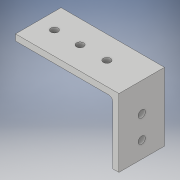
# Autodesk Inventor part: Right_BracketMount
Saved by Autodesk Inventor 2019 (Build 230136000, 136)
## iProperties
Created: 2019-05-22
Part Number: Right_BracketMount
Material: Generic
Document SubType Name: Modeling
Designer: Jorian Bruslind
Density: 1 g/cm^3
Appearance: Default
Author: Jorian Bruslind
Autodesk Inventor part; units mm, degrees
ref_plane "YZ Plane" through (0, 0, 0) normal (1, 0, 0) x (0, 1, 0)
ref_plane "XZ Plane" through (0, 0, 0) normal (0, 1, 0) x (-1, 0, 0)
ref_plane "XY Plane" through (0, 0, 0) normal (0, 0, 1) x (1, 0, 0)
sketch "Sketch1" plane through (0, 0, 0) normal (0, 1, 0) x (-1, 0, 0)
  line L0 (0, 0) -> (50, 0)
  line L1 (50, 0) -> (50, -22)
  line L2 (50, -22) -> (0, -22)
  line L3 (0, -22) -> (0, 0)
  dimension "d0" = 50
  dimension "d1" = 22
  constraints: 8 end point, 2 parallel, 1 horizontal, 1 perpendicular
  measures "d0" distance of L1.end L2.end
  measures "d1" distance of L0.end L1.end
extrude "Extrusion1" add sketch "Sketch1" along normal blind 3
sketch "Sketch2" plane through (0, 0, 0) normal (0, -1, 0) x (1, 0, 0)
  line L0 (-50, 0) -> (0, 0) projected
  line L1 (0, -22) -> (-50, -22) projected
  line L2 (0, 0) -> (-3, 0)
  line L3 (-3, 0) -> (-3, -22)
  line L4 (-3, -22) -> (0, -22)
  line L5 (0, -22) -> (0, 0)
  dimension "d4" = 3
  constraints: 8 end point, 2 parallel, 1 horizontal, 1 perpendicular, 1 point on line
  measures "d4" distance of L4.end L3.end
extrude "Extrusion2" add sketch "Sketch2" along normal blind 30
sketch "Sketch3" plane through (0, 3, 0) normal (0, 1, 0) x (1, 0, 0)
  circle A0 centre (-16.8, 11) radius 1.75
  line L0 (0, 22) -> (-50, 22) projected
  circle A1 centre (-42.2, 11) radius 1.75
  line L1 (-3, 0) -> (-29.8, 0)
  line L2 (-50, 0) -> (0, 0) projected
  line L3 (-29.8, 0) -> (-29.8, 11)
  circle A2 centre (-29.8, 11) radius 1.75
  dimension "d7" = 3.5
  dimension "d8" = 11
  dimension "d9" = 13.8
  dimension "d10" = 3.5
  dimension "d11" = 25.4
  dimension "d12" = 11
  dimension "d22" = 26.8
  dimension "d23" = 11
  dimension "d24" = 3.5
  constraints: 4 end point, 3 centre point, 1 coincident, 1 perpendicular, 1 point on line
  measures "d7" diameter of A0
  measures "d8" distance from line of L0 A0.centre
  measures "d9" horizontal distance of L1.start A0.centre
  measures "d10" diameter of A1
  measures "d11" distance of A0.centre A1.centre
  measures "d12" distance from line of L0 A1.centre
  measures "d22" distance of L1.start L1.end
  measures "d23" distance of L1.end L3.end
  measures "d24" diameter of A2
sketch "Sketch4" plane through (-3, 0, -22) normal (-1, 0, 0) x (0, 0, 1)
  line L0 (22, 0) -> (0, 0) projected
  line L1 (11, 0) -> (11, -11)
  circle A0 centre (11, -11) radius 1.75
  line L2 (11, -11) -> (11, -22)
  circle A1 centre (11, -22) radius 1.75
  dimension "d15" = 11
  dimension "d16" = 3.5
  dimension "d17" = 11
  dimension "d18" = 3.5
  constraints: 4 end point, 2 centre point, 2 coincident, 2 vertical, 1 midpoint
  measures "d15" distance of L1.start L1.end
  measures "d16" diameter of A0
  measures "d17" distance of L2.start L2.end
  measures "d18" diameter of A1
extrude "Extrusion4" cut sketch "Sketch4" against normal blind 3
fillet "Fillet1" radius 2 1 edges at (-3, 0, -11)
extrude "Extrusion5" cut sketch "Sketch3" against normal blind 3
body "Solid1"
